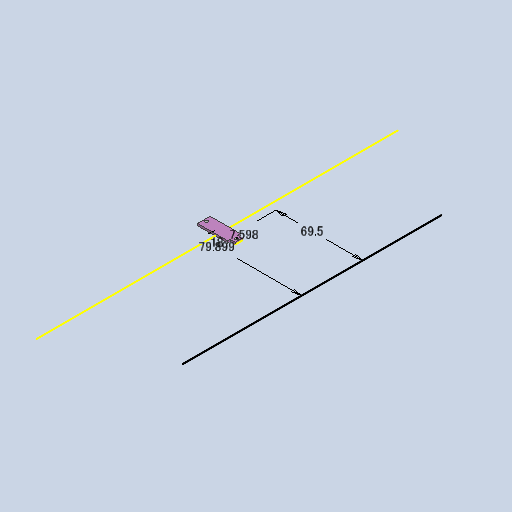
# Autodesk Inventor part: SideSensorCircuit
Saved by Autodesk Inventor 2025 (Build 290162000, 162)
## iProperties
Created: 2021-10-25
Part Number: SideSensorCircuit
Material: 一般
Document SubType Name: Modeling
Designer: shiok
Density: 1 g/cm^3
Appearance: 既定
Mass: 0.407924 g
Surface Area: 6.55632 cm^2
Volume: 0.407924 cm^3
Author: shiok
Autodesk Inventor part; units mm, degrees
ref_plane "YZ Plane" through (0, 0, 0) normal (1, 0, 0) x (0, 1, 0)
ref_plane "XZ Plane" through (0, 0, 0) normal (0, 1, 0) x (-1, 0, 0)
ref_plane "XY Plane" through (0, 0, 0) normal (0, 0, 1) x (1, 0, 0)
sketch "スケッチ1" plane through (0, 0, 0) normal (0, 1, 0) x (-1, 0, 0)
  line L0 (14, -5) -> (-14, -5)
  line L1 (-14, -5) -> (-14, 5)
  line L2 (-14, 5) -> (14, 5)
  line L3 (14, 5) -> (14, -5)
  line L4 (-14, 5) -> (14, -5) construction
  line L5 (14, 5) -> (-14, -5) construction
  point P0 (0, 0)
  point P1 (0, 0)
  dimension "d1" = 10
  dimension "d13" = 14
  constraints: 12 end point, 2 midpoint, 2 parallel, 1 coincident, 1 horizontal, 1 perpendicular
  measures "d1" distance of L0.end L1.end
  measures "d13" distance from line of L3 point (0, 0)
extrude "押し出し1" add sketch "スケッチ1" along normal blind 1.6
sketch "スケッチ3" plane through (0, 1.6, 0) normal (0, 1, 0) x (1, 0, 0)
  line L0 (14, -5) -> (14, 5) projected
  line L1 (14, 5) -> (10, 5)
  line L2 (10, 5) -> (10, 3)
  line L3 (10, 3) -> (14, 3)
  line L4 (14, 3) -> (14, 5)
  line L5 (-12.25, 0) -> (12.25, 0)
  line L6 (10, -5) -> (10, -3)
  line L7 (10, -3) -> (14, -3)
  line L8 (14, -5) -> (10, -5)
  line L9 (14, -3) -> (14, -5)
  point P0 (0, 0)
  dimension "d16" = 4
  dimension "d17" = 2
  constraints: 18 end point, 3 symmetric about line, 2 horizontal, 2 parallel, 1 perpendicular
  measures "d16" distance of L3.end L2.end
  measures "d17" distance of L2.end L1.end
extrude "押し出し2" cut sketch "スケッチ3" against normal blind 10
sketch "スケッチ4" plane through (0, 1.6, 0) normal (0, 1, 0) x (1, 0, 0)
  line L0 (10, 3) -> (10, 5) projected
  line L1 (10, -5) -> (10, -3) projected
  line L2 (10, 3) -> (10, -3)
  line L3 (10, 0) -> (14, 0)
  line L4 (14, -3) -> (14, 3) projected
  line L5 (-14, 5) -> (-14, -5) projected
  line L6 (-14, 0) -> (-12, 0)
  point P0 (0, 0)
  point P1 (12, 0)
  dimension "d27" = 2
  constraints: 6 end point, 4 midpoint, 1 coincident, 1 horizontal, 1 vertical
  measures "d27" distance of L6.start L6.end
hole "穴2" at (12, 1.6, 0) at (-12, 1.6, 0) direction (0, -1, 0) diameter 2.4 end through all clearance for "Countersunk Flat Head Screw ISO 2009/7046" size "M2" standard "ISO"
sketch "スケッチ7" plane through (0, 0, 0) normal (0, -1, 0) x (1, 0, 0)
  line L0 (75.7308, 106.5202) -> (76.0585, -99.7224)
  line L1 (75.7308, 106.5202) -> (76.0585, -99.7224)
  line L2 (0, 147.7687) -> (0, -140.9709) projected
  line L3 (75.7308, 106.5202) -> (76.0585, -99.7224)
  line L4 (14, 3) -> (14, -3) projected
  point P0 (0, 0)
  point P1 (6.4022, -1.407)
  point P2 (6.4022, -1.407)
  point P3 (-4, 0.784)
  dimension "d28" = 69.5
  dimension "d29" = 7.5978
  dimension "d31" = 18
  dimension "d32" = 79.8987
  constraints: 6 end point, 1 coincident, 9 other
  measures "d28" distance from line of L0 point (6.402, -1.407)
  measures "d29" distance from line of L4 point (6.402, -1.407)
  measures "d31" distance from line of L4 point (-4, 0.784)
  measures "d32" distance from line of L0 point (-4, 0.784)
